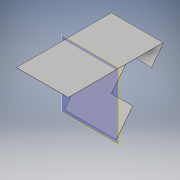
# Autodesk Inventor part: Autofeeder frame1
Saved by Autodesk Inventor 2016 (Build 200138000, 138)
## iProperties
Created: 2016-12-15
Part Number: Autofeeder frame1
Material: Generic
Document SubType Name: Sheet Metal
Designer: Student
Density: 1 g/cm^3
Sheet Metal Rule: Default_mm
Appearance: Default
Author: Student
Autodesk Inventor part; units mm, degrees
ref_plane "YZ Plane" through (0, 0, 0) normal (1, 0, 0) x (0, 1, 0)
ref_plane "XZ Plane" through (0, 0, 0) normal (0, 1, 0) x (-1, 0, 0)
ref_plane "XY Plane" through (0, 0, 0) normal (0, 0, 1) x (1, 0, 0)
sketch "Sketch1" plane through (0, 0, 0) normal (0, 1, 0) x (-1, 0, 0)
  line L0 (0, 0) -> (0, -228.6)
  line L1 (0, -228.6) -> (123.5964, -228.6)
  line L2 (123.5964, -228.6) -> (123.5964, 0)
  line L3 (123.5964, 0) -> (0, 0)
  dimension "d0" = 228.6
  dimension "d1" = 123.5964
  measures "d0" distance of L0.start L0.end
  measures "d1" distance of L0.end L1.end
extrude "Plate1" add sketch "Sketch1" along normal blind 0.5
sketch "Sketch2" plane through (0, 0.8078, -228.206) normal (0, -0.6156615, -0.7880108) x (1, 0, 0)
  line L0 (-123.5964, 0) -> (0, 0)
  line L1 (0, 0) -> (0, 184.15)
  line L2 (0, 184.15) -> (-123.5964, 184.15)
  line L3 (-123.5964, 184.15) -> (-123.5964, 0)
  constraints: 6 end point, 1 horizontal, 1 perpendicular, 1 vertical
edge flange "Flange1" height 184.15 angle 128 thickness 0.5 bend radius 0.5 thickness toward (0, -0.6156615, -0.7880108) relief tear relief width 0.5 relief depth 0.25 edges at (-61.7982, 0, -228.6) wall of the first edge with corners at (-123.5964, 0.8078, -228.206) (0, 0.8078, -228.206) (0, -144.3043, -114.8319) (-123.5964, -144.3043, -114.8319)
bend "Bend1"
corner "Corner1"
ref_plane "Work Plane2" through (-123.5964, 0, -114.3) normal (0, 0, -1) x (1, 0, 0)
ref_plane "Work Plane1" through (-123.5964, 0, 0) normal (0, 0, -1) x (1, 0, 0)
sketch "Sketch4" plane through (0, -144.6122, -115.2259) normal (0, -0.6156615, -0.7880108) x (-1, 0, 0)
  line L0 (0, 63.5) -> (50.8, 63.5)
  line L1 (50.8, 63.5) -> (50.8, 136.271)
  line L2 (50.8, 136.271) -> (0, 136.271)
  line L3 (0, 0) -> (0, 182.0997) projected
  line L4 (0, 63.5) -> (0, 136.271)
  line L5 (123.5964, 0) -> (0, 0) projected
  dimension "d22" = 50.8
  dimension "d23" = 63.5
  dimension "d24" = 72.771
  constraints: 8 end point, 2 perpendicular, 1 collinear, 1 horizontal, 1 point on line
  measures "d22" distance of L0.start L0.end
  measures "d23" distance between parallel lines of L5 L0
  measures "d24" distance between parallel lines of L0 L2
extrude "Cut2" cut sketch "Sketch4" against normal blind 0.5
equation "\"d25\" = Thickness"
equation "\"d3\" = BendReliefWidth"
equation "\"d4\" = BendReliefDepth"
equation "\"d5\" = MinimumRemnant"
equation "\"d6\" = BendRadius"
equation "\"d9\" = BendRadius"
equation "\"d10\" = CornerReliefSize"
equation "\"d11\" = GapSize"
equation "\"d12\" = JacobiRadiusSize"
equation "\"BendRadius\" = Thickness"
equation "\"BendReliefWidth\" = Thickness"
equation "\"BendReliefDepth\" = 0.5 * Thickness"
equation "\"CornerReliefSize\" = 4 * Thickness"
equation "\"MinimumRemnant\" = 2 * Thickness"
equation "\"TransitionRadius\" = BendRadius"
equation "\"JacobiRadiusSize\" = BendRadius"
equation "\"GapSize\" = Thickness"
equation "\"d2\" = BendRadius"
equation "\"Thickness\" = 0.5"
body "Solid1"
